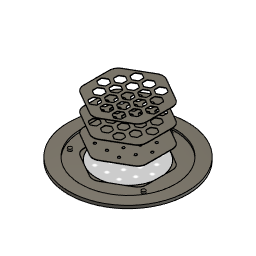
Shadow.Mask.Kit (Autodesk Fusion 360 design; units mm, degrees)
Autodesk Fusion 360 part; units mm, degrees
(part 1 of 2)
sketch "Stencil.Full.Hex" plane through (0, 0, 0) normal (0, 1, 0) x (1, 0, 0)
  circle A0 centre (0, 0) radius 39
  line L0 (0, 0) -> (0, -4.25) construction
  line L1 (0, 0) -> (3.6806, -2.125) construction
  line L2 (0, 0) -> (3.6806, 2.125) construction
  line L3 (0, 0) -> (0, 4.25) construction
  line L4 (0, 0) -> (-3.6806, 2.125) construction
  line L5 (0, 0) -> (-3.6806, -2.125) construction
  line L6 (0.5, -3.9613) -> (3.1806, -2.4137)
  line L7 (3.6806, -1.5476) -> (3.6806, 1.5476)
  line L8 (3.1806, 2.4137) -> (0.5, 3.9613)
  line L9 (-0.5, 3.9613) -> (-3.1806, 2.4137)
  line L10 (-3.6806, 1.5476) -> (-3.6806, -1.5476)
  line L11 (-3.1806, -2.4137) -> (-0.5, -3.9613)
  arc A1 (-3.6806, -1.5476) -> (-3.1806, -2.4137) centre (-2.6806, -1.5476) ccw
  arc A2 (-0.5, -3.9613) -> (0.5, -3.9613) centre (0, -3.0953) ccw
  arc A3 (3.1806, -2.4137) -> (3.6806, -1.5476) centre (2.6806, -1.5476) ccw
  arc A4 (3.6806, 1.5476) -> (3.1806, 2.4137) centre (2.6806, 1.5476) ccw
  arc A5 (0.5, 3.9613) -> (-0.5, 3.9613) centre (0, 3.0953) ccw
  arc A6 (-3.1806, 2.4137) -> (-3.6806, 1.5476) centre (-2.6806, 1.5476) ccw
  line L12 (-10, -17.32) -> (-13.6806, -15.195) construction
  line L13 (-13.6806, -15.7724) -> (-13.6806, -18.8676)
  line L14 (-6.8194, -14.9063) -> (-9.5, -13.3587)
  line L15 (-10, -17.32) -> (-6.3194, -19.445) construction
  line L16 (-10, -17.32) -> (-10, -21.57) construction
  line L17 (-10, -17.32) -> (-10, -13.07) construction
  line L18 (-13.1806, -19.7337) -> (-10.5, -21.2813)
  line L19 (-10, -17.32) -> (-13.6806, -19.445) construction
  arc A7 (-9.5, -13.3587) -> (-10.5, -13.3587) centre (-10, -14.2247) ccw
  line L20 (-10, -17.32) -> (-6.3194, -15.195) construction
  line L21 (-6.3194, -18.8676) -> (-6.3194, -15.7724)
  arc A8 (-6.8194, -19.7337) -> (-6.3194, -18.8676) centre (-7.3194, -18.8676) ccw
  line L22 (-9.5, -21.2813) -> (-6.8194, -19.7337)
  arc A9 (-13.1806, -14.9063) -> (-13.6806, -15.7724) centre (-12.6806, -15.7724) ccw
  arc A10 (-13.6806, -18.8676) -> (-13.1806, -19.7337) centre (-12.6806, -18.8676) ccw
  line L23 (-10.5, -13.3587) -> (-13.1806, -14.9063)
  arc A11 (-10.5, -21.2813) -> (-9.5, -21.2813) centre (-10, -20.4153) ccw
  arc A12 (-6.3194, -15.7724) -> (-6.8194, -14.9063) centre (-7.3194, -15.7724) ccw
  line L24 (0, -17.32) -> (-3.6806, -15.195) construction
  line L25 (-3.6806, -15.7724) -> (-3.6806, -18.8676)
  line L26 (3.1806, -14.9063) -> (0.5, -13.3587)
  line L27 (0, -17.32) -> (3.6806, -19.445) construction
  line L28 (0, -17.32) -> (0, -21.57) construction
  line L29 (0, -17.32) -> (0, -13.07) construction
  line L30 (-3.1806, -19.7337) -> (-0.5, -21.2813)
  line L31 (0, -17.32) -> (-3.6806, -19.445) construction
  arc A13 (0.5, -13.3587) -> (-0.5, -13.3587) centre (0, -14.2247) ccw
  line L32 (0, -17.32) -> (3.6806, -15.195) construction
  line L33 (3.6806, -18.8676) -> (3.6806, -15.7724)
  arc A14 (3.1806, -19.7337) -> (3.6806, -18.8676) centre (2.6806, -18.8676) ccw
  line L34 (0.5, -21.2813) -> (3.1806, -19.7337)
  arc A15 (-3.1806, -14.9063) -> (-3.6806, -15.7724) centre (-2.6806, -15.7724) ccw
  arc A16 (-3.6806, -18.8676) -> (-3.1806, -19.7337) centre (-2.6806, -18.8676) ccw
  line L35 (-0.5, -13.3587) -> (-3.1806, -14.9063)
  arc A17 (-0.5, -21.2813) -> (0.5, -21.2813) centre (0, -20.4153) ccw
  arc A18 (3.6806, -15.7724) -> (3.1806, -14.9063) centre (2.6806, -15.7724) ccw
  line L36 (10, -17.32) -> (6.3194, -15.195) construction
  line L37 (6.3194, -15.7724) -> (6.3194, -18.8676)
  line L38 (13.1806, -14.9063) -> (10.5, -13.3587)
  line L39 (10, -17.32) -> (13.6806, -19.445) construction
  line L40 (10, -17.32) -> (10, -21.57) construction
  line L41 (10, -17.32) -> (10, -13.07) construction
  line L42 (6.8194, -19.7337) -> (9.5, -21.2813)
  line L43 (10, -17.32) -> (6.3194, -19.445) construction
  arc A19 (10.5, -13.3587) -> (9.5, -13.3587) centre (10, -14.2247) ccw
  line L44 (10, -17.32) -> (13.6806, -15.195) construction
  line L45 (13.6806, -18.8676) -> (13.6806, -15.7724)
  arc A20 (13.1806, -19.7337) -> (13.6806, -18.8676) centre (12.6806, -18.8676) ccw
  line L46 (10.5, -21.2813) -> (13.1806, -19.7337)
  arc A21 (6.8194, -14.9063) -> (6.3194, -15.7724) centre (7.3194, -15.7724) ccw
  arc A22 (6.3194, -18.8676) -> (6.8194, -19.7337) centre (7.3194, -18.8676) ccw
  line L47 (9.5, -13.3587) -> (6.8194, -14.9063)
  arc A23 (9.5, -21.2813) -> (10.5, -21.2813) centre (10, -20.4153) ccw
  arc A24 (13.6806, -15.7724) -> (13.1806, -14.9063) centre (12.6806, -15.7724) ccw
  line L48 (-20, 0) -> (-23.6806, 2.125) construction
  line L49 (-23.6806, 1.5476) -> (-23.6806, -1.5476)
  line L50 (-16.8194, 2.4137) -> (-19.5, 3.9613)
  line L51 (-20, 0) -> (-16.3194, -2.125) construction
  line L52 (-20, 0) -> (-20, -4.25) construction
  line L53 (-20, 0) -> (-20, 4.25) construction
  line L54 (-23.1806, -2.4137) -> (-20.5, -3.9613)
  line L55 (-20, 0) -> (-23.6806, -2.125) construction
  arc A25 (-19.5, 3.9613) -> (-20.5, 3.9613) centre (-20, 3.0953) ccw
  line L56 (-20, 0) -> (-16.3194, 2.125) construction
  line L57 (-16.3194, -1.5476) -> (-16.3194, 1.5476)
  arc A26 (-16.8194, -2.4137) -> (-16.3194, -1.5476) centre (-17.3194, -1.5476) ccw
  line L58 (-19.5, -3.9613) -> (-16.8194, -2.4137)
  arc A27 (-23.1806, 2.4137) -> (-23.6806, 1.5476) centre (-22.6806, 1.5476) ccw
  arc A28 (-23.6806, -1.5476) -> (-23.1806, -2.4137) centre (-22.6806, -1.5476) ccw
  line L59 (-20.5, 3.9613) -> (-23.1806, 2.4137)
  arc A29 (-20.5, -3.9613) -> (-19.5, -3.9613) centre (-20, -3.0953) ccw
  arc A30 (-16.3194, 1.5476) -> (-16.8194, 2.4137) centre (-17.3194, 1.5476) ccw
  line L60 (-10, 0) -> (-13.6806, 2.125) construction
  line L61 (-13.6806, 1.5476) -> (-13.6806, -1.5476)
  line L62 (-6.8194, 2.4137) -> (-9.5, 3.9613)
  line L63 (-10, 0) -> (-6.3194, -2.125) construction
  line L64 (-10, 0) -> (-10, -4.25) construction
  line L65 (-10, 0) -> (-10, 4.25) construction
  line L66 (-13.1806, -2.4137) -> (-10.5, -3.9613)
  line L67 (-10, 0) -> (-13.6806, -2.125) construction
  arc A31 (-9.5, 3.9613) -> (-10.5, 3.9613) centre (-10, 3.0953) ccw
  line L68 (-10, 0) -> (-6.3194, 2.125) construction
  line L69 (-6.3194, -1.5476) -> (-6.3194, 1.5476)
  arc A32 (-6.8194, -2.4137) -> (-6.3194, -1.5476) centre (-7.3194, -1.5476) ccw
  line L70 (-9.5, -3.9613) -> (-6.8194, -2.4137)
  arc A33 (-13.1806, 2.4137) -> (-13.6806, 1.5476) centre (-12.6806, 1.5476) ccw
  arc A34 (-13.6806, -1.5476) -> (-13.1806, -2.4137) centre (-12.6806, -1.5476) ccw
  line L71 (-10.5, 3.9613) -> (-13.1806, 2.4137)
  arc A35 (-10.5, -3.9613) -> (-9.5, -3.9613) centre (-10, -3.0953) ccw
  arc A36 (-6.3194, 1.5476) -> (-6.8194, 2.4137) centre (-7.3194, 1.5476) ccw
  line L72 (10, 0) -> (6.3194, 2.125) construction
  line L73 (6.3194, 1.5476) -> (6.3194, -1.5476)
  line L74 (13.1806, 2.4137) -> (10.5, 3.9613)
  line L75 (10, 0) -> (13.6806, -2.125) construction
  line L76 (10, 0) -> (10, -4.25) construction
  line L77 (10, 0) -> (10, 4.25) construction
  line L78 (6.8194, -2.4137) -> (9.5, -3.9613)
  line L79 (10, 0) -> (6.3194, -2.125) construction
  arc A37 (10.5, 3.9613) -> (9.5, 3.9613) centre (10, 3.0953) ccw
  line L80 (10, 0) -> (13.6806, 2.125) construction
  line L81 (13.6806, -1.5476) -> (13.6806, 1.5476)
  arc A38 (13.1806, -2.4137) -> (13.6806, -1.5476) centre (12.6806, -1.5476) ccw
  line L82 (10.5, -3.9613) -> (13.1806, -2.4137)
  arc A39 (6.8194, 2.4137) -> (6.3194, 1.5476) centre (7.3194, 1.5476) ccw
  arc A40 (6.3194, -1.5476) -> (6.8194, -2.4137) centre (7.3194, -1.5476) ccw
  line L83 (9.5, 3.9613) -> (6.8194, 2.4137)
  arc A41 (9.5, -3.9613) -> (10.5, -3.9613) centre (10, -3.0953) ccw
  arc A42 (13.6806, 1.5476) -> (13.1806, 2.4137) centre (12.6806, 1.5476) ccw
  line L84 (20, 0) -> (16.3194, 2.125) construction
  line L85 (16.3194, 1.5476) -> (16.3194, -1.5476)
  line L86 (23.1806, 2.4137) -> (20.5, 3.9613)
  line L87 (20, 0) -> (23.6806, -2.125) construction
  line L88 (20, 0) -> (20, -4.25) construction
  line L89 (20, 0) -> (20, 4.25) construction
  line L90 (16.8194, -2.4137) -> (19.5, -3.9613)
  line L91 (20, 0) -> (16.3194, -2.125) construction
  arc A43 (20.5, 3.9613) -> (19.5, 3.9613) centre (20, 3.0953) ccw
  line L92 (20, 0) -> (23.6806, 2.125) construction
  line L93 (23.6806, -1.5476) -> (23.6806, 1.5476)
  arc A44 (23.1806, -2.4137) -> (23.6806, -1.5476) centre (22.6806, -1.5476) ccw
  line L94 (20.5, -3.9613) -> (23.1806, -2.4137)
  arc A45 (16.8194, 2.4137) -> (16.3194, 1.5476) centre (17.3194, 1.5476) ccw
  arc A46 (16.3194, -1.5476) -> (16.8194, -2.4137) centre (17.3194, -1.5476) ccw
  line L95 (19.5, 3.9613) -> (16.8194, 2.4137)
  arc A47 (19.5, -3.9613) -> (20.5, -3.9613) centre (20, -3.0953) ccw
  arc A48 (23.6806, 1.5476) -> (23.1806, 2.4137) centre (22.6806, 1.5476) ccw
  line L96 (-10, 17.32) -> (-13.6806, 19.445) construction
  line L97 (-13.6806, 18.8676) -> (-13.6806, 15.7724)
  line L98 (-6.8194, 19.7337) -> (-9.5, 21.2813)
  line L99 (-10, 17.32) -> (-6.3194, 15.195) construction
  line L100 (-10, 17.32) -> (-10, 13.07) construction
  line L101 (-10, 17.32) -> (-10, 21.57) construction
  line L102 (-13.1806, 14.9063) -> (-10.5, 13.3587)
  line L103 (-10, 17.32) -> (-13.6806, 15.195) construction
  arc A49 (-9.5, 21.2813) -> (-10.5, 21.2813) centre (-10, 20.4153) ccw
  line L104 (-10, 17.32) -> (-6.3194, 19.445) construction
  line L105 (-6.3194, 15.7724) -> (-6.3194, 18.8676)
  arc A50 (-6.8194, 14.9063) -> (-6.3194, 15.7724) centre (-7.3194, 15.7724) ccw
  line L106 (-9.5, 13.3587) -> (-6.8194, 14.9063)
  arc A51 (-13.1806, 19.7337) -> (-13.6806, 18.8676) centre (-12.6806, 18.8676) ccw
  arc A52 (-13.6806, 15.7724) -> (-13.1806, 14.9063) centre (-12.6806, 15.7724) ccw
  line L107 (-10.5, 21.2813) -> (-13.1806, 19.7337)
  arc A53 (-10.5, 13.3587) -> (-9.5, 13.3587) centre (-10, 14.2247) ccw
  arc A54 (-6.3194, 18.8676) -> (-6.8194, 19.7337) centre (-7.3194, 18.8676) ccw
  line L108 (0, 17.32) -> (-3.6806, 19.445) construction
  line L109 (-3.6806, 18.8676) -> (-3.6806, 15.7724)
  line L110 (3.1806, 19.7337) -> (0.5, 21.2813)
  line L111 (0, 17.32) -> (3.6806, 15.195) construction
  line L112 (0, 17.32) -> (0, 13.07) construction
  line L113 (0, 17.32) -> (0, 21.57) construction
  line L114 (-3.1806, 14.9063) -> (-0.5, 13.3587)
  line L115 (0, 17.32) -> (-3.6806, 15.195) construction
  arc A55 (0.5, 21.2813) -> (-0.5, 21.2813) centre (0, 20.4153) ccw
  line L116 (0, 17.32) -> (3.6806, 19.445) construction
  line L117 (3.6806, 15.7724) -> (3.6806, 18.8676)
  arc A56 (3.1806, 14.9063) -> (3.6806, 15.7724) centre (2.6806, 15.7724) ccw
  line L118 (0.5, 13.3587) -> (3.1806, 14.9063)
  arc A57 (-3.1806, 19.7337) -> (-3.6806, 18.8676) centre (-2.6806, 18.8676) ccw
  arc A58 (-3.6806, 15.7724) -> (-3.1806, 14.9063) centre (-2.6806, 15.7724) ccw
  line L119 (-0.5, 21.2813) -> (-3.1806, 19.7337)
  arc A59 (-0.5, 13.3587) -> (0.5, 13.3587) centre (0, 14.2247) ccw
  arc A60 (3.6806, 18.8676) -> (3.1806, 19.7337) centre (2.6806, 18.8676) ccw
  line L120 (10, 17.32) -> (6.3194, 19.445) construction
  line L121 (6.3194, 18.8676) -> (6.3194, 15.7724)
  line L122 (13.1806, 19.7337) -> (10.5, 21.2813)
  line L123 (10, 17.32) -> (13.6806, 15.195) construction
  line L124 (10, 17.32) -> (10, 13.07) construction
  line L125 (10, 17.32) -> (10, 21.57) construction
  line L126 (6.8194, 14.9063) -> (9.5, 13.3587)
  line L127 (10, 17.32) -> (6.3194, 15.195) construction
  arc A61 (10.5, 21.2813) -> (9.5, 21.2813) centre (10, 20.4153) ccw
  line L128 (10, 17.32) -> (13.6806, 19.445) construction
  line L129 (13.6806, 15.7724) -> (13.6806, 18.8676)
  arc A62 (13.1806, 14.9063) -> (13.6806, 15.7724) centre (12.6806, 15.7724) ccw
  line L130 (10.5, 13.3587) -> (13.1806, 14.9063)
  arc A63 (6.8194, 19.7337) -> (6.3194, 18.8676) centre (7.3194, 18.8676) ccw
  arc A64 (6.3194, 15.7724) -> (6.8194, 14.9063) centre (7.3194, 15.7724) ccw
  line L131 (9.5, 21.2813) -> (6.8194, 19.7337)
  arc A65 (9.5, 13.3587) -> (10.5, 13.3587) centre (10, 14.2247) ccw
  arc A66 (13.6806, 18.8676) -> (13.1806, 19.7337) centre (12.6806, 18.8676) ccw
  arc A67 (8.1806, 6.2466) -> (8.6806, 7.1126) centre (7.6806, 7.1126) ccw
  arc A68 (8.6806, 10.2079) -> (8.1806, 11.0739) centre (7.6806, 10.2079) ccw
  line L132 (5, 8.6603) -> (1.3194, 6.5353) construction
  line L133 (8.1806, 11.0739) -> (5.5, 12.6216)
  line L134 (5, 8.6603) -> (8.6806, 6.5353) construction
  arc A69 (4.5, 4.6989) -> (5.5, 4.6989) centre (5, 5.565) ccw
  arc A70 (1.8194, 11.0739) -> (1.3194, 10.2079) centre (2.3194, 10.2079) ccw
  line L135 (5, 8.6603) -> (1.3194, 10.7853) construction
  line L136 (4.5, 12.6216) -> (1.8194, 11.0739)
  line L137 (8.6806, 7.1126) -> (8.6806, 10.2079)
  line L138 (5, 8.6603) -> (8.6806, 10.7853) construction
  line L139 (5, 8.6603) -> (5, 4.4103) construction
  line L140 (1.3194, 10.2079) -> (1.3194, 7.1126)
  line L141 (1.8194, 6.2466) -> (4.5, 4.6989)
  arc A71 (1.3194, 7.1126) -> (1.8194, 6.2466) centre (2.3194, 7.1126) ccw
  line L142 (5.5, 4.6989) -> (8.1806, 6.2466)
  arc A72 (5.5, 12.6216) -> (4.5, 12.6216) centre (5, 11.7556) ccw
  line L143 (5, 8.6603) -> (5, 12.9103) construction
  arc A73 (-1.3194, 10.2079) -> (-1.8194, 11.0739) centre (-2.3194, 10.2079) ccw
  arc A74 (-4.5, 12.6216) -> (-5.5, 12.6216) centre (-5, 11.7556) ccw
  line L144 (-5, 8.6603) -> (-5, 4.4103) construction
  line L145 (-5.5, 12.6216) -> (-8.1806, 11.0739)
  line L146 (-5, 8.6603) -> (-1.3194, 10.7853) construction
  arc A75 (-1.8194, 6.2466) -> (-1.3194, 7.1126) centre (-2.3194, 7.1126) ccw
  arc A76 (-8.6806, 7.1126) -> (-8.1806, 6.2466) centre (-7.6806, 7.1126) ccw
  line L147 (-5, 8.6603) -> (-8.6806, 6.5353) construction
  line L148 (-8.6806, 10.2079) -> (-8.6806, 7.1126)
  line L149 (-1.8194, 11.0739) -> (-4.5, 12.6216)
  line L150 (-5, 8.6603) -> (-5, 12.9103) construction
  line L151 (-5, 8.6603) -> (-1.3194, 6.5353) construction
  line L152 (-8.1806, 6.2466) -> (-5.5, 4.6989)
  line L153 (-4.5, 4.6989) -> (-1.8194, 6.2466)
  arc A77 (-5.5, 4.6989) -> (-4.5, 4.6989) centre (-5, 5.565) ccw
  line L154 (-1.3194, 7.1126) -> (-1.3194, 10.2079)
  arc A78 (-8.1806, 11.0739) -> (-8.6806, 10.2079) centre (-7.6806, 10.2079) ccw
  line L155 (-5, 8.6603) -> (-8.6806, 10.7853) construction
  arc A79 (-9.5, 3.9613) -> (-10.5, 3.9613) centre (-10, 3.0953) ccw
  arc A80 (-13.1806, 2.4137) -> (-13.6806, 1.5476) centre (-12.6806, 1.5476) ccw
  line L156 (-10, 0) -> (-6.3194, -2.125) construction
  line L157 (-13.6806, 1.5476) -> (-13.6806, -1.5476)
  line L158 (-10, 0) -> (-10, 4.25) construction
  arc A81 (-6.3194, 1.5476) -> (-6.8194, 2.4137) centre (-7.3194, 1.5476) ccw
  arc A82 (-10.5, -3.9613) -> (-9.5, -3.9613) centre (-10, -3.0953) ccw
  line L159 (-10, 0) -> (-10, -4.25) construction
  line L160 (-13.1806, -2.4137) -> (-10.5, -3.9613)
  line L161 (-10.5, 3.9613) -> (-13.1806, 2.4137)
  line L162 (-10, 0) -> (-13.6806, 2.125) construction
  line L163 (-10, 0) -> (-6.3194, 2.125) construction
  line L164 (-9.5, -3.9613) -> (-6.8194, -2.4137)
  line L165 (-6.3194, -1.5476) -> (-6.3194, 1.5476)
  arc A83 (-6.8194, -2.4137) -> (-6.3194, -1.5476) centre (-7.3194, -1.5476) ccw
  line L166 (-6.8194, 2.4137) -> (-9.5, 3.9613)
  arc A84 (-13.6806, -1.5476) -> (-13.1806, -2.4137) centre (-12.6806, -1.5476) ccw
  line L167 (-10, 0) -> (-13.6806, -2.125) construction
  arc A85 (-8.1806, -6.2466) -> (-8.6806, -7.1126) centre (-7.6806, -7.1126) ccw
  arc A86 (-8.6806, -10.2079) -> (-8.1806, -11.0739) centre (-7.6806, -10.2079) ccw
  line L168 (-5, -8.6603) -> (-1.3194, -6.5353) construction
  line L169 (-8.1806, -11.0739) -> (-5.5, -12.6216)
  line L170 (-5, -8.6603) -> (-8.6806, -6.5353) construction
  arc A87 (-4.5, -4.6989) -> (-5.5, -4.6989) centre (-5, -5.565) ccw
  arc A88 (-1.8194, -11.0739) -> (-1.3194, -10.2079) centre (-2.3194, -10.2079) ccw
  line L171 (-5, -8.6603) -> (-1.3194, -10.7853) construction
  line L172 (-4.5, -12.6216) -> (-1.8194, -11.0739)
  line L173 (-8.6806, -7.1126) -> (-8.6806, -10.2079)
  line L174 (-5, -8.6603) -> (-8.6806, -10.7853) construction
  line L175 (-5, -8.6603) -> (-5, -4.4103) construction
  line L176 (-1.3194, -10.2079) -> (-1.3194, -7.1126)
  line L177 (-1.8194, -6.2466) -> (-4.5, -4.6989)
  arc A89 (-1.3194, -7.1126) -> (-1.8194, -6.2466) centre (-2.3194, -7.1126) ccw
  line L178 (-5.5, -4.6989) -> (-8.1806, -6.2466)
  arc A90 (-5.5, -12.6216) -> (-4.5, -12.6216) centre (-5, -11.7556) ccw
  line L179 (-5, -8.6603) -> (-5, -12.9103) construction
  arc A91 (1.3194, -10.2079) -> (1.8194, -11.0739) centre (2.3194, -10.2079) ccw
  arc A92 (4.5, -12.6216) -> (5.5, -12.6216) centre (5, -11.7556) ccw
  line L180 (5, -8.6603) -> (5, -4.4103) construction
  line L181 (5.5, -12.6216) -> (8.1806, -11.0739)
  line L182 (5, -8.6603) -> (1.3194, -10.7853) construction
  arc A93 (1.8194, -6.2466) -> (1.3194, -7.1126) centre (2.3194, -7.1126) ccw
  arc A94 (8.6806, -7.1126) -> (8.1806, -6.2466) centre (7.6806, -7.1126) ccw
  line L183 (5, -8.6603) -> (8.6806, -6.5353) construction
  line L184 (8.6806, -10.2079) -> (8.6806, -7.1126)
  line L185 (1.8194, -11.0739) -> (4.5, -12.6216)
  line L186 (5, -8.6603) -> (5, -12.9103) construction
  line L187 (5, -8.6603) -> (1.3194, -6.5353) construction
  line L188 (8.1806, -6.2466) -> (5.5, -4.6989)
  line L189 (4.5, -4.6989) -> (1.8194, -6.2466)
  arc A95 (5.5, -4.6989) -> (4.5, -4.6989) centre (5, -5.565) ccw
  line L190 (1.3194, -7.1126) -> (1.3194, -10.2079)
  arc A96 (8.1806, -11.0739) -> (8.6806, -10.2079) centre (7.6806, -10.2079) ccw
  line L191 (5, -8.6603) -> (8.6806, -10.7853) construction
  line L192 (11.8194, 6.2466) -> (14.5, 4.6989)
  line L193 (15, 8.6603) -> (11.3194, 10.7853) construction
  arc A97 (18.6806, 10.2079) -> (18.1806, 11.0739) centre (17.6806, 10.2079) ccw
  line L194 (15, 8.6603) -> (18.6806, 6.5353) construction
  line L195 (15, 8.6603) -> (18.6806, 10.7853) construction
  arc A98 (11.3194, 7.1126) -> (11.8194, 6.2466) centre (12.3194, 7.1126) ccw
  line L196 (15, 8.6603) -> (15, 4.4103) construction
  line L197 (15, 8.6603) -> (11.3194, 6.5353) construction
  arc A99 (11.8194, 11.0739) -> (11.3194, 10.2079) centre (12.3194, 10.2079) ccw
  arc A100 (18.1806, 6.2466) -> (18.6806, 7.1126) centre (17.6806, 7.1126) ccw
  line L198 (18.1806, 11.0739) -> (15.5, 12.6216)
  line L199 (18.6806, 7.1126) -> (18.6806, 10.2079)
  line L200 (11.3194, 10.2079) -> (11.3194, 7.1126)
  line L201 (15.5, 4.6989) -> (18.1806, 6.2466)
  line L202 (15, 8.6603) -> (15, 12.9103) construction
  line L203 (14.5, 12.6216) -> (11.8194, 11.0739)
  arc A101 (15.5, 12.6216) -> (14.5, 12.6216) centre (15, 11.7556) ccw
  arc A102 (14.5, 4.6989) -> (15.5, 4.6989) centre (15, 5.565) ccw
  arc A103 (-11.8194, 6.2466) -> (-11.3194, 7.1126) centre (-12.3194, 7.1126) ccw
  arc A104 (-18.6806, 7.1126) -> (-18.1806, 6.2466) centre (-17.6806, 7.1126) ccw
  arc A105 (-15.5, 4.6989) -> (-14.5, 4.6989) centre (-15, 5.565) ccw
  line L204 (-15, 8.6603) -> (-15, 12.9103) construction
  line L205 (-11.3194, 7.1126) -> (-11.3194, 10.2079)
  line L206 (-15, 8.6603) -> (-18.6806, 10.7853) construction
  line L207 (-15, 8.6603) -> (-18.6806, 6.5353) construction
  arc A106 (-18.1806, 11.0739) -> (-18.6806, 10.2079) centre (-17.6806, 10.2079) ccw
  line L208 (-18.1806, 6.2466) -> (-15.5, 4.6989)
  arc A107 (-14.5, 12.6216) -> (-15.5, 12.6216) centre (-15, 11.7556) ccw
  line L209 (-15.5, 12.6216) -> (-18.1806, 11.0739)
  line L210 (-15, 8.6603) -> (-11.3194, 6.5353) construction
  arc A108 (-11.3194, 10.2079) -> (-11.8194, 11.0739) centre (-12.3194, 10.2079) ccw
  line L211 (-14.5, 4.6989) -> (-11.8194, 6.2466)
  line L212 (-11.8194, 11.0739) -> (-14.5, 12.6216)
  line L213 (-15, 8.6603) -> (-11.3194, 10.7853) construction
  line L214 (-15, 8.6603) -> (-15, 4.4103) construction
  line L215 (-18.6806, 10.2079) -> (-18.6806, 7.1126)
  arc A109 (15.5, -4.6989) -> (14.5, -4.6989) centre (15, -5.565) ccw
  arc A110 (11.8194, -6.2466) -> (11.3194, -7.1126) centre (12.3194, -7.1126) ccw
  line L216 (15, -8.6603) -> (18.6806, -10.7853) construction
  line L217 (15, -8.6603) -> (15, -12.9103) construction
  line L218 (11.8194, -11.0739) -> (14.5, -12.6216)
  arc A111 (18.6806, -7.1126) -> (18.1806, -6.2466) centre (17.6806, -7.1126) ccw
  line L219 (14.5, -4.6989) -> (11.8194, -6.2466)
  line L220 (15, -8.6603) -> (11.3194, -10.7853) construction
  arc A112 (11.3194, -10.2079) -> (11.8194, -11.0739) centre (12.3194, -10.2079) ccw
  line L221 (18.1806, -6.2466) -> (15.5, -4.6989)
  line L222 (15, -8.6603) -> (15, -4.4103) construction
  arc A113 (18.1806, -11.0739) -> (18.6806, -10.2079) centre (17.6806, -10.2079) ccw
  line L223 (15, -8.6603) -> (11.3194, -6.5353) construction
  line L224 (15.5, -12.6216) -> (18.1806, -11.0739)
  line L225 (18.6806, -10.2079) -> (18.6806, -7.1126)
  arc A114 (14.5, -12.6216) -> (15.5, -12.6216) centre (15, -11.7556) ccw
  line L226 (15, -8.6603) -> (18.6806, -6.5353) construction
  line L227 (11.3194, -7.1126) -> (11.3194, -10.2079)
  line L228 (-18.1806, -11.0739) -> (-15.5, -12.6216)
  line L229 (-11.3194, -10.2079) -> (-11.3194, -7.1126)
  arc A115 (-18.6806, -10.2079) -> (-18.1806, -11.0739) centre (-17.6806, -10.2079) ccw
  line L230 (-15, -8.6603) -> (-11.3194, -6.5353) construction
  line L231 (-14.5, -12.6216) -> (-11.8194, -11.0739)
  line L232 (-18.6806, -7.1126) -> (-18.6806, -10.2079)
  line L233 (-15, -8.6603) -> (-15, -4.4103) construction
  line L234 (-15, -8.6603) -> (-18.6806, -10.7853) construction
  arc A116 (-15.5, -12.6216) -> (-14.5, -12.6216) centre (-15, -11.7556) ccw
  line L235 (-15, -8.6603) -> (-11.3194, -10.7853) construction
  line L236 (-15, -8.6603) -> (-15, -12.9103) construction
  line L237 (-15, -8.6603) -> (-18.6806, -6.5353) construction
  arc A117 (-18.1806, -6.2466) -> (-18.6806, -7.1126) centre (-17.6806, -7.1126) ccw
  line L238 (-15.5, -4.6989) -> (-18.1806, -6.2466)
  arc A118 (-14.5, -4.6989) -> (-15.5, -4.6989) centre (-15, -5.565) ccw
  arc A119 (-11.8194, -11.0739) -> (-11.3194, -10.2079) centre (-12.3194, -10.2079) ccw
  line L239 (-11.8194, -6.2466) -> (-14.5, -4.6989)
  arc A120 (-11.3194, -7.1126) -> (-11.8194, -6.2466) centre (-12.3194, -7.1126) ccw
  circle A121 centre (0, 0) radius 30
  line L240 (0, 0) -> (0, 35) construction
  circle A122 centre (0, 35) radius 1.5
  circle A123 centre (-30.3109, -17.5) radius 1.5
  circle A124 centre (30.3109, -17.5) radius 1.5
  line L241 (3.75, -27.8349) -> (22.2308, -17.1651)
  line L242 (25.9808, -10.6699) -> (25.9808, 10.6699)
  line L243 (22.2308, 17.1651) -> (3.75, 27.8349)
  line L244 (-3.75, 27.8349) -> (-22.2308, 17.1651)
  line L245 (-25.9808, 10.6699) -> (-25.9808, -10.6699)
  line L246 (-22.2308, -17.1651) -> (-3.75, -27.8349)
  arc A125 (-22.2308, 17.1651) -> (-25.9808, 10.6699) centre (-18.4808, 10.6699) ccw
  arc A126 (3.75, 27.8349) -> (-3.75, 27.8349) centre (0, 21.3397) ccw
  arc A127 (25.9808, 10.6699) -> (22.2308, 17.1651) centre (18.4808, 10.6699) ccw
  arc A128 (22.2308, -17.1651) -> (25.9808, -10.6699) centre (18.4808, -10.6699) ccw
  arc A129 (-3.75, -27.8349) -> (3.75, -27.8349) centre (0, -21.3397) ccw
  arc A130 (-25.9808, -10.6699) -> (-22.2308, -17.1651) centre (-18.4808, -10.6699) ccw
  circle A131 centre (0, 0) radius 25.9808
  circle A132 centre (0, 0) radius 49
  circle A133 centre (0, 0) radius 1
  circle A134 centre (10, 0) radius 1
  circle A135 centre (5, 8.6603) radius 1
  circle A136 centre (-5, 8.6603) radius 1
  circle A137 centre (-10, 0) radius 1
  circle A138 centre (-5, -8.6603) radius 1
  circle A139 centre (5, -8.6603) radius 1
  circle A140 centre (20, 0) radius 1
  circle A141 centre (10, 17.3205) radius 1
  circle A142 centre (-10, 17.3205) radius 1
  circle A143 centre (-20, 0) radius 1
  circle A144 centre (-10, -17.3205) radius 1
  circle A145 centre (10, -17.3205) radius 1
  circle A146 centre (15, 8.6603) radius 1
  circle A147 centre (0, 17.3205) radius 1
  circle A148 centre (-15, 8.6603) radius 1
  circle A149 centre (-15, -8.6603) radius 1
  circle A150 centre (0, -17.3205) radius 1
  circle A151 centre (15, -8.6603) radius 1
  line L247 (-9.5, 13.6092) -> (-7.0359, 15.0318)
  line L248 (-6.5359, 15.8979) -> (-6.5359, 18.7432)
  line L249 (-7.0359, 19.6092) -> (-9.5, 21.0318)
  line L250 (-10.5, 21.0318) -> (-12.9641, 19.6092)
  line L251 (-13.4641, 18.7432) -> (-13.4641, 15.8979)
  line L252 (-12.9641, 15.0318) -> (-10.5, 13.6092)
  line L253 (0.5, 13.6092) -> (2.9641, 15.0318)
  line L254 (3.4641, 15.8979) -> (3.4641, 18.7432)
  line L255 (2.9641, 19.6092) -> (0.5, 21.0318)
  line L256 (-0.5, 21.0318) -> (-2.9641, 19.6092)
  line L257 (-3.4641, 18.7432) -> (-3.4641, 15.8979)
  line L258 (-2.9641, 15.0318) -> (-0.5, 13.6092)
  line L259 (10.5, 13.6087) -> (12.9641, 15.0313)
  line L260 (13.4641, 15.8974) -> (13.4641, 18.7426)
  line L261 (12.9641, 19.6087) -> (10.5, 21.0313)
  line L262 (9.5, 21.0313) -> (7.0359, 19.6087)
  line L263 (6.5359, 18.7426) -> (6.5359, 15.8974)
  line L264 (7.0359, 15.0313) -> (9.5, 13.6087)
  line L265 (-14.5, 4.9489) -> (-12.0359, 6.3716)
  line L266 (-11.5359, 7.2376) -> (-11.5359, 10.0829)
  line L267 (-12.0359, 10.9489) -> (-14.5, 12.3716)
  line L268 (-15.5, 12.3716) -> (-17.9641, 10.9489)
  line L269 (-18.4641, 10.0829) -> (-18.4641, 7.2376)
  line L270 (-17.9641, 6.3716) -> (-15.5, 4.9489)
  line L271 (-4.5, 4.9489) -> (-2.0359, 6.3716)
  line L272 (-1.5359, 7.2376) -> (-1.5359, 10.0829)
  line L273 (-2.0359, 10.9489) -> (-4.5, 12.3716)
  line L274 (-5.5, 12.3716) -> (-7.9641, 10.9489)
  line L275 (-8.4641, 10.0829) -> (-8.4641, 7.2376)
  line L276 (-7.9641, 6.3716) -> (-5.5, 4.9489)
  line L277 (5.5, 4.9489) -> (7.9641, 6.3716)
  line L278 (8.4641, 7.2376) -> (8.4641, 10.0829)
  line L279 (7.9641, 10.9489) -> (5.5, 12.3716)
  line L280 (4.5, 12.3716) -> (2.0359, 10.9489)
  line L281 (1.5359, 10.0829) -> (1.5359, 7.2376)
  line L282 (2.0359, 6.3716) -> (4.5, 4.9489)
  line L283 (15.5, 4.9489) -> (17.9641, 6.3716)
  line L284 (18.4641, 7.2376) -> (18.4641, 10.0829)
  line L285 (17.9641, 10.9489) -> (15.5, 12.3716)
  line L286 (14.5, 12.3716) -> (12.0359, 10.9489)
  line L287 (11.5359, 10.0829) -> (11.5359, 7.2376)
  line L288 (12.0359, 6.3716) -> (14.5, 4.9489)
  line L289 (-19.5, -3.7113) -> (-17.0359, -2.2887)
  line L290 (-16.5359, -1.4226) -> (-16.5359, 1.4226)
  line L291 (-17.0359, 2.2887) -> (-19.5, 3.7113)
  line L292 (-20.5, 3.7113) -> (-22.9641, 2.2887)
  line L293 (-23.4641, 1.4226) -> (-23.4641, -1.4226)
  line L294 (-22.9641, -2.2887) -> (-20.5, -3.7113)
  line L295 (-9.5, -3.7113) -> (-7.0359, -2.2887)
  line L296 (-6.5359, -1.4226) -> (-6.5359, 1.4226)
  line L297 (-7.0359, 2.2887) -> (-9.5, 3.7113)
  line L298 (-10.5, 3.7113) -> (-12.9641, 2.2887)
  line L299 (-13.4641, 1.4226) -> (-13.4641, -1.4226)
  line L300 (-12.9641, -2.2887) -> (-10.5, -3.7113)
  line L301 (0.5, -3.7113) -> (2.9641, -2.2887)
  line L302 (3.4641, -1.4226) -> (3.4641, 1.4226)
  line L303 (2.9641, 2.2887) -> (0.5, 3.7113)
  line L304 (-0.5, 3.7113) -> (-2.9641, 2.2887)
  line L305 (-3.4641, 1.4226) -> (-3.4641, -1.4226)
  line L306 (-2.9641, -2.2887) -> (-0.5, -3.7113)
  line L307 (10.5, -3.7113) -> (12.9641, -2.2887)
  line L308 (13.4641, -1.4226) -> (13.4641, 1.4226)
  line L309 (12.9641, 2.2887) -> (10.5, 3.7113)
  line L310 (9.5, 3.7113) -> (7.0359, 2.2887)
  line L311 (6.5359, 1.4226) -> (6.5359, -1.4226)
  line L312 (7.0359, -2.2887) -> (9.5, -3.7113)
  line L313 (20.5, -3.7113) -> (22.9641, -2.2887)
  line L314 (23.4641, -1.4226) -> (23.4641, 1.4226)
  line L315 (22.9641, 2.2887) -> (20.5, 3.7113)
  line L316 (19.5, 3.7113) -> (17.0359, 2.2887)
  line L317 (16.5359, 1.4226) -> (16.5359, -1.4226)
  line L318 (17.0359, -2.2887) -> (19.5, -3.7113)
  line L319 (-14.5, -12.3716) -> (-12.0359, -10.9489)
  line L320 (-11.5359, -10.0829) -> (-11.5359, -7.2376)
  line L321 (-12.0359, -6.3716) -> (-14.5, -4.9489)
  line L322 (-15.5, -4.9489) -> (-17.9641, -6.3716)
  line L323 (-18.4641, -7.2376) -> (-18.4641, -10.0829)
  line L324 (-17.9641, -10.9489) -> (-15.5, -12.3716)
  line L325 (-4.5, -12.3716) -> (-2.0359, -10.9489)
  line L326 (-1.5359, -10.0829) -> (-1.5359, -7.2376)
  line L327 (-2.0359, -6.3716) -> (-4.5, -4.9489)
  line L328 (-5.5, -4.9489) -> (-7.9641, -6.3716)
  line L329 (-8.4641, -7.2376) -> (-8.4641, -10.0829)
  line L330 (-7.9641, -10.9489) -> (-5.5, -12.3716)
  line L331 (5.5, -12.3716) -> (7.9641, -10.9489)
  line L332 (8.4641, -10.0829) -> (8.4641, -7.2376)
  line L333 (7.9641, -6.3716) -> (5.5, -4.9489)
  line L334 (4.5, -4.9489) -> (2.0359, -6.3716)
  line L335 (1.5359, -7.2376) -> (1.5359, -10.0829)
  line L336 (2.0359, -10.9489) -> (4.5, -12.3716)
  line L337 (15.5, -12.3716) -> (17.9641, -10.9489)
  line L338 (18.4641, -10.0829) -> (18.4641, -7.2376)
  line L339 (17.9641, -6.3716) -> (15.5, -4.9489)
  line L340 (14.5, -4.9489) -> (12.0359, -6.3716)
  line L341 (11.5359, -7.2376) -> (11.5359, -10.0829)
  line L342 (12.0359, -10.9489) -> (14.5, -12.3716)
  line L343 (-9.5, -21.0313) -> (-7.0359, -19.6087)
  line L344 (-6.5359, -18.7426) -> (-6.5359, -15.8974)
  line L345 (-7.0359, -15.0313) -> (-9.5, -13.6087)
  line L346 (-10.5, -13.6087) -> (-12.9641, -15.0313)
  line L347 (-13.4641, -15.8974) -> (-13.4641, -18.7426)
  line L348 (-12.9641, -19.6087) -> (-10.5, -21.0313)
  line L349 (0.5, -21.0318) -> (2.9641, -19.6092)
  line L350 (3.4641, -18.7432) -> (3.4641, -15.8979)
  line L351 (2.9641, -15.0318) -> (0.5, -13.6092)
  line L352 (-0.5, -13.6092) -> (-2.9641, -15.0318)
  line L353 (-3.4641, -15.8979) -> (-3.4641, -18.7432)
  line L354 (-2.9641, -19.6092) -> (-0.5, -21.0318)
  line L355 (10.5, -21.0313) -> (12.9641, -19.6087)
  line L356 (13.4641, -18.7426) -> (13.4641, -15.8974)
  line L357 (12.9641, -15.0313) -> (10.5, -13.6087)
  line L358 (9.5, -13.6087) -> (7.0359, -15.0313)
  line L359 (6.5359, -15.8974) -> (6.5359, -18.7426)
  line L360 (7.0359, -19.6087) -> (9.5, -21.0313)
  arc A152 (-12.9641, 19.6092) -> (-13.4641, 18.7432) centre (-12.4641, 18.7432) ccw
  arc A153 (-9.5, 21.0318) -> (-10.5, 21.0318) centre (-10, 20.1658) ccw
  arc A154 (-6.5359, 18.7432) -> (-7.0359, 19.6092) centre (-7.5359, 18.7432) ccw
  arc A155 (-7.0359, 15.0318) -> (-6.5359, 15.8979) centre (-7.5359, 15.8979) ccw
  arc A156 (-10.5, 13.6092) -> (-9.5, 13.6092) centre (-10, 14.4752) ccw
  arc A157 (-13.4641, 15.8979) -> (-12.9641, 15.0318) centre (-12.4641, 15.8979) ccw
  arc A158 (-2.9641, 19.6092) -> (-3.4641, 18.7432) centre (-2.4641, 18.7432) ccw
  arc A159 (0.5, 21.0318) -> (-0.5, 21.0318) centre (0, 20.1658) ccw
  arc A160 (3.4641, 18.7432) -> (2.9641, 19.6092) centre (2.4641, 18.7432) ccw
  arc A161 (2.9641, 15.0318) -> (3.4641, 15.8979) centre (2.4641, 15.8979) ccw
  arc A162 (-0.5, 13.6092) -> (0.5, 13.6092) centre (0, 14.4752) ccw
  arc A163 (-3.4641, 15.8979) -> (-2.9641, 15.0318) centre (-2.4641, 15.8979) ccw
  arc A164 (6.5359, 15.8974) -> (7.0359, 15.0313) centre (7.5359, 15.8974) ccw
  arc A165 (7.0359, 19.6087) -> (6.5359, 18.7426) centre (7.5359, 18.7426) ccw
  arc A166 (10.5, 21.0313) -> (9.5, 21.0313) centre (10, 20.1653) ccw
  arc A167 (13.4641, 18.7426) -> (12.9641, 19.6087) centre (12.4641, 18.7426) ccw
  arc A168 (9.5, 13.6087) -> (10.5, 13.6087) centre (10, 14.4747) ccw
  arc A169 (12.9641, 15.0313) -> (13.4641, 15.8974) centre (12.4641, 15.8974) ccw
  arc A170 (-14.5, 12.3716) -> (-15.5, 12.3716) centre (-15, 11.5056) ccw
  arc A171 (-11.5359, 10.0829) -> (-12.0359, 10.9489) centre (-12.5359, 10.0829) ccw
  arc A172 (-12.0359, 6.3716) -> (-11.5359, 7.2376) centre (-12.5359, 7.2376) ccw
  arc A173 (-15.5, 4.9489) -> (-14.5, 4.9489) centre (-15, 5.815) ccw
  arc A174 (-18.4641, 7.2376) -> (-17.9641, 6.3716) centre (-17.4641, 7.2376) ccw
  arc A175 (-17.9641, 10.9489) -> (-18.4641, 10.0829) centre (-17.4641, 10.0829) ccw
  arc A176 (-4.5, 12.3716) -> (-5.5, 12.3716) centre (-5, 11.5056) ccw
  arc A177 (-1.5359, 10.0829) -> (-2.0359, 10.9489) centre (-2.5359, 10.0829) ccw
  arc A178 (-2.0359, 6.3716) -> (-1.5359, 7.2376) centre (-2.5359, 7.2376) ccw
  arc A179 (-5.5, 4.9489) -> (-4.5, 4.9489) centre (-5, 5.815) ccw
  arc A180 (-8.4641, 7.2376) -> (-7.9641, 6.3716) centre (-7.4641, 7.2376) ccw
  arc A181 (-7.9641, 10.9489) -> (-8.4641, 10.0829) centre (-7.4641, 10.0829) ccw
  arc A182 (2.0359, 10.9489) -> (1.5359, 10.0829) centre (2.5359, 10.0829) ccw
  arc A183 (5.5, 12.3716) -> (4.5, 12.3716) centre (5, 11.5056) ccw
  arc A184 (8.4641, 10.0829) -> (7.9641, 10.9489) centre (7.4641, 10.0829) ccw
  arc A185 (7.9641, 6.3716) -> (8.4641, 7.2376) centre (7.4641, 7.2376) ccw
  arc A186 (4.5, 4.9489) -> (5.5, 4.9489) centre (5, 5.815) ccw
  arc A187 (1.5359, 7.2376) -> (2.0359, 6.3716) centre (2.5359, 7.2376) ccw
  arc A188 (15.5, 12.3716) -> (14.5, 12.3716) centre (15, 11.5056) ccw
  arc A189 (18.4641, 10.0829) -> (17.9641, 10.9489) centre (17.4641, 10.0829) ccw
  arc A190 (17.9641, 6.3716) -> (18.4641, 7.2376) centre (17.4641, 7.2376) ccw
  arc A191 (14.5, 4.9489) -> (15.5, 4.9489) centre (15, 5.815) ccw
  arc A192 (11.5359, 7.2376) -> (12.0359, 6.3716) centre (12.5359, 7.2376) ccw
  arc A193 (12.0359, 10.9489) -> (11.5359, 10.0829) centre (12.5359, 10.0829) ccw
  arc A194 (20.5, 3.7113) -> (19.5, 3.7113) centre (20, 2.8453) ccw
  arc A195 (23.4641, 1.4226) -> (22.9641, 2.2887) centre (22.4641, 1.4226) ccw
  arc A196 (22.9641, -2.2887) -> (23.4641, -1.4226) centre (22.4641, -1.4226) ccw
  arc A197 (19.5, -3.7113) -> (20.5, -3.7113) centre (20, -2.8453) ccw
  arc A198 (16.5359, -1.4226) -> (17.0359, -2.2887) centre (17.5359, -1.4226) ccw
  arc A199 (17.0359, 2.2887) -> (16.5359, 1.4226) centre (17.5359, 1.4226) ccw
  arc A200 (13.4641, 1.4226) -> (12.9641, 2.2887) centre (12.4641, 1.4226) ccw
  arc A201 (12.9641, -2.2887) -> (13.4641, -1.4226) centre (12.4641, -1.4226) ccw
  arc A202 (9.5, -3.7113) -> (10.5, -3.7113) centre (10, -2.8453) ccw
  arc A203 (6.5359, -1.4226) -> (7.0359, -2.2887) centre (7.5359, -1.4226) ccw
  arc A204 (7.0359, 2.2887) -> (6.5359, 1.4226) centre (7.5359, 1.4226) ccw
  arc A205 (10.5, 3.7113) -> (9.5, 3.7113) centre (10, 2.8453) ccw
  arc A206 (3.4641, 1.4226) -> (2.9641, 2.2887) centre (2.4641, 1.4226) ccw
  arc A207 (0.5, 3.7113) -> (-0.5, 3.7113) centre (0, 2.8453) ccw
  arc A208 (-2.9641, 2.2887) -> (-3.4641, 1.4226) centre (-2.4641, 1.4226) ccw
  arc A209 (-3.4641, -1.4226) -> (-2.9641, -2.2887) centre (-2.4641, -1.4226) ccw
  arc A210 (-0.5, -3.7113) -> (0.5, -3.7113) centre (0, -2.8453) ccw
  arc A211 (2.9641, -2.2887) -> (3.4641, -1.4226) centre (2.4641, -1.4226) ccw
  arc A212 (-6.5359, 1.4226) -> (-7.0359, 2.2887) centre (-7.5359, 1.4226) ccw
  arc A213 (-9.5, 3.7113) -> (-10.5, 3.7113) centre (-10, 2.8453) ccw
  arc A214 (-12.9641, 2.2887) -> (-13.4641, 1.4226) centre (-12.4641, 1.4226) ccw
  arc A215 (-13.4641, -1.4226) -> (-12.9641, -2.2887) centre (-12.4641, -1.4226) ccw
  arc A216 (-10.5, -3.7113) -> (-9.5, -3.7113) centre (-10, -2.8453) ccw
  arc A217 (-7.0359, -2.2887) -> (-6.5359, -1.4226) centre (-7.5359, -1.4226) ccw
  arc A218 (-16.5359, 1.4226) -> (-17.0359, 2.2887) centre (-17.5359, 1.4226) ccw
  arc A219 (-19.5, 3.7113) -> (-20.5, 3.7113) centre (-20, 2.8453) ccw
  arc A220 (-22.9641, 2.2887) -> (-23.4641, 1.4226) centre (-22.4641, 1.4226) ccw
  arc A221 (-14.5, -4.9489) -> (-15.5, -4.9489) centre (-15, -5.815) ccw
  arc A222 (-11.5359, -7.2376) -> (-12.0359, -6.3716) centre (-12.5359, -7.2376) ccw
  arc A223 (-12.0359, -10.9489) -> (-11.5359, -10.0829) centre (-12.5359, -10.0829) ccw
  arc A224 (-15.5, -12.3716) -> (-14.5, -12.3716) centre (-15, -11.5056) ccw
  arc A225 (-18.4641, -10.0829) -> (-17.9641, -10.9489) centre (-17.4641, -10.0829) ccw
  arc A226 (-17.9641, -6.3716) -> (-18.4641, -7.2376) centre (-17.4641, -7.2376) ccw
  arc A227 (-7.9641, -6.3716) -> (-8.4641, -7.2376) centre (-7.4641, -7.2376) ccw
  arc A228 (-4.5, -4.9489) -> (-5.5, -4.9489) centre (-5, -5.815) ccw
  arc A229 (-1.5359, -7.2376) -> (-2.0359, -6.3716) centre (-2.5359, -7.2376) ccw
  arc A230 (-2.0359, -10.9489) -> (-1.5359, -10.0829) centre (-2.5359, -10.0829) ccw
  arc A231 (-5.5, -12.3716) -> (-4.5, -12.3716) centre (-5, -11.5056) ccw
  arc A232 (-8.4641, -10.0829) -> (-7.9641, -10.9489) centre (-7.4641, -10.0829) ccw
  arc A233 (2.0359, -6.3716) -> (1.5359, -7.2376) centre (2.5359, -7.2376) ccw
  arc A234 (5.5, -4.9489) -> (4.5, -4.9489) centre (5, -5.815) ccw
  arc A235 (8.4641, -7.2376) -> (7.9641, -6.3716) centre (7.4641, -7.2376) ccw
  arc A236 (7.9641, -10.9489) -> (8.4641, -10.0829) centre (7.4641, -10.0829) ccw
  arc A237 (4.5, -12.3716) -> (5.5, -12.3716) centre (5, -11.5056) ccw
  arc A238 (1.5359, -10.0829) -> (2.0359, -10.9489) centre (2.5359, -10.0829) ccw
  arc A239 (12.0359, -6.3716) -> (11.5359, -7.2376) centre (12.5359, -7.2376) ccw
  arc A240 (15.5, -4.9489) -> (14.5, -4.9489) centre (15, -5.815) ccw
  arc A241 (18.4641, -7.2376) -> (17.9641, -6.3716) centre (17.4641, -7.2376) ccw
  arc A242 (17.9641, -10.9489) -> (18.4641, -10.0829) centre (17.4641, -10.0829) ccw
  arc A243 (14.5, -12.3716) -> (15.5, -12.3716) centre (15, -11.5056) ccw
  arc A244 (11.5359, -10.0829) -> (12.0359, -10.9489) centre (12.5359, -10.0829) ccw
  arc A245 (-12.9641, -15.0313) -> (-13.4641, -15.8974) centre (-12.4641, -15.8974) ccw
  arc A246 (-9.5, -13.6087) -> (-10.5, -13.6087) centre (-10, -14.4747) ccw
  arc A247 (-6.5359, -15.8974) -> (-7.0359, -15.0313) centre (-7.5359, -15.8974) ccw
  arc A248 (-7.0359, -19.6087) -> (-6.5359, -18.7426) centre (-7.5359, -18.7426) ccw
  arc A249 (-10.5, -21.0313) -> (-9.5, -21.0313) centre (-10, -20.1653) ccw
  arc A250 (-13.4641, -18.7426) -> (-12.9641, -19.6087) centre (-12.4641, -18.7426) ccw
  arc A251 (-3.4641, -18.7432) -> (-2.9641, -19.6092) centre (-2.4641, -18.7432) ccw
  arc A252 (-2.9641, -15.0318) -> (-3.4641, -15.8979) centre (-2.4641, -15.8979) ccw
  arc A253 (0.5, -13.6092) -> (-0.5, -13.6092) centre (0, -14.4752) ccw
  arc A254 (3.4641, -15.8979) -> (2.9641, -15.0318) centre (2.4641, -15.8979) ccw
  arc A255 (2.9641, -19.6092) -> (3.4641, -18.7432) centre (2.4641, -18.7432) ccw
  arc A256 (-0.5, -21.0318) -> (0.5, -21.0318) centre (0, -20.1658) ccw
  arc A257 (10.5, -13.6087) -> (9.5, -13.6087) centre (10, -14.4747) ccw
  arc A258 (7.0359, -15.0313) -> (6.5359, -15.8974) centre (7.5359, -15.8974) ccw
  arc A259 (6.5359, -18.7426) -> (7.0359, -19.6087) centre (7.5359, -18.7426) ccw
  arc A260 (9.5, -21.0313) -> (10.5, -21.0313) centre (10, -20.1653) ccw
  arc A261 (12.9641, -19.6087) -> (13.4641, -18.7426) centre (12.4641, -18.7426) ccw
  arc A262 (13.4641, -15.8974) -> (12.9641, -15.0313) centre (12.4641, -15.8974) ccw
  arc A263 (-23.4641, -1.4226) -> (-22.9641, -2.2887) centre (-22.4641, -1.4226) ccw
  arc A264 (-20.5, -3.7113) -> (-19.5, -3.7113) centre (-20, -2.8453) ccw
  arc A265 (-17.0359, -2.2887) -> (-16.5359, -1.4226) centre (-17.5359, -1.4226) ccw
  point P0 (-10, -17.32)
  point P1 (-10, -17.32)
  point P2 (-10, -17.32)
  point P3 (0, -17.32)
  point P4 (0, -17.32)
  point P5 (0, -17.32)
  point P6 (10, -17.32)
  point P7 (10, -17.32)
  point P8 (10, -17.32)
  point P9 (-20, 0)
  point P10 (-20, 0)
  point P11 (-20, 0)
  point P12 (-10, 0)
  point P13 (-10, 0)
  point P14 (-10, 0)
  point P15 (10, 0)
  point P16 (10, 0)
  point P17 (10, 0)
  point P18 (20, 0)
  point P19 (20, 0)
  point P20 (20, 0)
  point P21 (-10, 17.32)
  point P22 (-10, 17.32)
  point P23 (-10, 17.32)
  point P24 (0, 17.32)
  point P25 (0, 17.32)
  point P26 (0, 17.32)
  point P27 (10, 17.32)
  point P28 (10, 17.32)
  point P29 (10, 17.32)
  point P30 (5, 8.6603)
  point P31 (5, 8.6603)
  point P32 (5, 8.6603)
  point P33 (-5, 8.6603)
  point P34 (-5, 8.6603)
  point P35 (-5, 8.6603)
  point P36 (-10, 0)
  point P37 (-10, 0)
  point P38 (-10, 0)
  point P39 (-5, -8.6603)
  point P40 (-5, -8.6603)
  point P41 (-5, -8.6603)
  point P42 (5, -8.6603)
  point P43 (5, -8.6603)
  point P44 (5, -8.6603)
  point P45 (15, 8.6603)
  point P46 (15, 8.6603)
  point P47 (15, 8.6603)
  point P48 (-15, 8.6603)
  point P49 (-15, 8.6603)
  point P50 (-15, 8.6603)
  point P51 (15, -8.6603)
  point P52 (15, -8.6603)
  point P53 (15, -8.6603)
  point P54 (-15, -8.6603)
  point P55 (-15, -8.6603)
  point P56 (-15, -8.6603)
  point P57 (-10, 17.3205)
  point P58 (0, 13.3205)
  point P59 (0, 17.3205)
  point P60 (10, 13.32)
  point P61 (10, 17.32)
  point P62 (-15, 4.6603)
  point P63 (-15, 8.6603)
  point P64 (-5, 4.6603)
  point P65 (-5, 8.6603)
  point P66 (5, 4.6603)
  point P67 (5, 8.6603)
  point P68 (15, 4.6603)
  point P69 (15, 8.6603)
  point P70 (-20, -4)
  point P71 (-20, 0)
  point P72 (-10, -4)
  point P73 (-10, 0)
  point P74 (0, -4)
  point P75 (10, -4)
  point P76 (10, 0)
  point P77 (20, -4)
  point P78 (20, 0)
  point P79 (-15, -12.6603)
  point P80 (-15, -8.6603)
  point P81 (-5, -12.6603)
  point P82 (-5, -8.6603)
  point P83 (5, -12.6603)
  point P84 (5, -8.6603)
  point P85 (15, -12.6603)
  point P86 (15, -8.6603)
  point P87 (-10, -21.32)
  point P88 (-10, -17.32)
  point P89 (0, -21.3205)
  point P90 (0, -17.3205)
  point P91 (10, -21.32)
  point P92 (10, -17.32)
  dimension "d1" = 78
  dimension "d3" = 4.25
  dimension "d5" = 360
  dimension "d6" = 1
  dimension "d7" = 1
  dimension "d8" = 1
  dimension "d11" = 10
  dimension "d12" = 17.32
  dimension "d14" = 360
  dimension "d17" = 10
  dimension "d18" = 0
  dimension "d21" = -10
  dimension "d22" = 0
  dimension "d25" = 10
  dimension "d26" = 0
  dimension "d29" = -10
  dimension "d30" = 0
  dimension "d31" = 60
  dimension "d34" = 35
  dimension "d36" = 3
  dimension "d38" = 360
  dimension "d39" = 7.5
  dimension "d52" = 98
  dimension "d55" = 2
  dimension "d56" = 2
  dimension "d58" = 360
  dimension "d59" = 2
  dimension "d61" = 360
  dimension "d62" = 2
  dimension "d64" = 360
  dimension "d68" = 4
  dimension "d69" = 4
  dimension "d70" = 4
  dimension "d71" = 4
  dimension "d72" = 4
  dimension "d73" = 4
  dimension "d74" = 4
  dimension "d75" = 4
  dimension "d76" = 4
  dimension "d77" = 4
  dimension "d78" = 4
  dimension "d79" = 4
  dimension "d80" = 4
  dimension "d81" = 4
  dimension "d82" = 4
  dimension "d83" = 4
  dimension "d84" = 4
  dimension "d85" = 4
  dimension "d86" = 1
  dimension "d87" = 1
  constraint coincident A0.centre L0.start
  constraint vertical L0
  constraint tangent L10 A1
  constraint tangent L11 A1
  constraint tangent L11 A2
  constraint tangent L6 A2
  constraint tangent L6 A3
  constraint tangent L7 A3
  constraint equal A2 A3
  constraint tangent L7 A4
  constraint tangent L8 A4
  constraint tangent L9 A5
  constraint tangent L8 A5
  constraint equal A4 A5
  constraint tangent L10 A6
  constraint tangent L9 A6
  constraint equal A4 A6
  constraint vertical L240
  constraint coincident L240.end A122.centre
  constraint tangent L245 A125
  constraint tangent L244 A125
  constraint tangent L244 A126
  constraint tangent L243 A126
  constraint equal A125 A126
  constraint tangent L243 A127
  constraint tangent L242 A127
  constraint equal A125 A127
  constraint tangent L242 A128
  constraint tangent L241 A128
  constraint equal A125 A128
  constraint tangent L241 A129
  constraint tangent L246 A129
  constraint equal A125 A129
  constraint tangent L246 A130
  constraint tangent L245 A130
  constraint equal A125 A130
  constraint tangent L242 A131
  constraint coincident P76 P17
  constraint coincident P78 P20
  constraint coincident P69 P47
  constraint coincident P57 A142.centre
  constraint coincident L112 P58
  constraint coincident P59 A147.centre
  constraint coincident L124 P60
  constraint coincident P61 P29
  constraint coincident L214 P62
  constraint coincident P63 P50
  constraint coincident P65 P35
  constraint coincident L144 P64
  constraint coincident L139 P66
  constraint coincident P67 P32
  constraint coincident L196 P68
  constraint coincident P71 P11
  constraint coincident L52 P70
  constraint coincident P73 P38
  constraint coincident L64 P72
  constraint coincident L0 P74
  constraint coincident L76 P75
  constraint coincident L88 P77
  constraint coincident L236 P79
  constraint coincident P80 P56
  constraint coincident L179 P81
  constraint coincident P82 P41
  constraint coincident P84 P44
  constraint coincident L186 P83
  constraint coincident L217 P85
  constraint coincident P86 P53
  constraint coincident L16 P87
  constraint coincident P88 P2
  constraint coincident L28 P89
  constraint coincident P90 A150.centre
  constraint coincident L40 P91
  constraint coincident P92 P8
  constraint tangent L251 A152
  constraint tangent L250 A152
  constraint tangent L250 A153
  constraint tangent L249 A153
  constraint equal A152 A153
  constraint tangent L249 A154
  constraint tangent L248 A154
  constraint equal A152 A154
  constraint tangent L248 A155
  constraint tangent L247 A155
  constraint equal A152 A155
  constraint tangent L247 A156
  constraint tangent L252 A156
  constraint equal A152 A156
  constraint tangent L252 A157
  constraint tangent L251 A157
  constraint equal A152 A157
  constraint tangent L257 A158
  constraint tangent L256 A158
  constraint equal A152 A158
  constraint tangent L256 A159
  constraint tangent L255 A159
  constraint equal A152 A159
  constraint tangent L255 A160
  constraint tangent L254 A160
  constraint equal A152 A160
  constraint tangent L254 A161
  constraint tangent L253 A161
  constraint equal A152 A161
  constraint coincident P58 L253
  constraint coincident P58 L258
  constraint tangent L253 A162
  constraint tangent L258 A162
  constraint equal A152 A162
  constraint tangent L258 A163
  constraint tangent L257 A163
  constraint equal A152 A163
  constraint tangent L264 A164
  constraint tangent L263 A164
  constraint equal A152 A164
  constraint tangent L263 A165
  constraint tangent L262 A165
  constraint equal A152 A165
  constraint tangent L262 A166
  constraint tangent L261 A166
  constraint equal A152 A166
  constraint tangent L261 A167
  constraint tangent L260 A167
  constraint equal A152 A167
  constraint coincident P60 L264
  constraint coincident P60 L259
  constraint tangent L264 A168
  constraint tangent L259 A168
  constraint equal A152 A168
  constraint tangent L260 A169
  constraint tangent L259 A169
  constraint equal A152 A169
  constraint tangent L268 A170
  constraint tangent L267 A170
  constraint equal A152 A170
  constraint tangent L267 A171
  constraint tangent L266 A171
  constraint equal A152 A171
  constraint tangent L266 A172
  constraint tangent L265 A172
  constraint equal A152 A172
  constraint coincident P62 L265
  constraint coincident P62 L270
  constraint tangent L265 A173
  constraint tangent L270 A173
  constraint equal A152 A173
  constraint tangent L270 A174
  constraint tangent L269 A174
  constraint equal A152 A174
  constraint tangent L268 A175
  constraint tangent L269 A175
  constraint equal A152 A175
  constraint tangent L274 A176
  constraint tangent L273 A176
  constraint equal A152 A176
  constraint tangent L273 A177
  constraint tangent L272 A177
  constraint equal A152 A177
  constraint tangent L272 A178
  constraint tangent L271 A178
  constraint equal A152 A178
  constraint coincident P64 L271
  constraint coincident P64 L276
  constraint tangent L271 A179
  constraint tangent L276 A179
  constraint equal A152 A179
  constraint tangent L276 A180
  constraint tangent L275 A180
  constraint equal A152 A180
  constraint tangent L275 A181
  constraint tangent L274 A181
  constraint equal A152 A181
  constraint tangent L281 A182
  constraint tangent L280 A182
  constraint equal A152 A182
  constraint tangent L280 A183
  constraint tangent L279 A183
  constraint equal A152 A183
  constraint tangent L279 A184
  constraint tangent L278 A184
  constraint equal A152 A184
  constraint tangent L278 A185
  constraint tangent L277 A185
  constraint equal A152 A185
  constraint coincident P66 L277
  constraint coincident P66 L282
  constraint tangent L277 A186
  constraint tangent L282 A186
  constraint equal A152 A186
  constraint tangent L282 A187
  constraint tangent L281 A187
  constraint equal A152 A187
  constraint tangent L286 A188
  constraint tangent L285 A188
  constraint equal A152 A188
  constraint tangent L285 A189
  constraint tangent L284 A189
  constraint equal A152 A189
  constraint tangent L284 A190
  constraint tangent L283 A190
  constraint equal A152 A190
  constraint coincident P68 L288
  constraint coincident P68 L283
  constraint tangent L288 A191
  constraint tangent L283 A191
  constraint equal A152 A191
  constraint tangent L288 A192
  constraint tangent L287 A192
  constraint equal A152 A192
  constraint tangent L287 A193
  constraint tangent L286 A193
  constraint equal A152 A193
  constraint tangent L316 A194
  constraint tangent L315 A194
  constraint equal A152 A194
  constraint tangent L315 A195
  constraint tangent L314 A195
  constraint equal A152 A195
  constraint tangent L314 A196
  constraint tangent L313 A196
  constraint equal A152 A196
  constraint coincident P77 L313
  constraint coincident P77 L318
  constraint tangent L313 A197
  constraint tangent L318 A197
  constraint equal A152 A197
  constraint tangent L318 A198
  constraint tangent L317 A198
  constraint equal A152 A198
  constraint tangent L317 A199
  constraint tangent L316 A199
  constraint equal A152 A199
  constraint tangent L309 A200
  constraint tangent L308 A200
  constraint equal A152 A200
  constraint tangent L308 A201
  constraint tangent L307 A201
  constraint equal A152 A201
  constraint coincident P75 L307
  constraint coincident P75 L312
  constraint tangent L307 A202
  constraint tangent L312 A202
  constraint equal A152 A202
  constraint tangent L312 A203
  constraint tangent L311 A203
  constraint equal A152 A203
  constraint tangent L311 A204
  constraint tangent L310 A204
  constraint equal A152 A204
  constraint tangent L310 A205